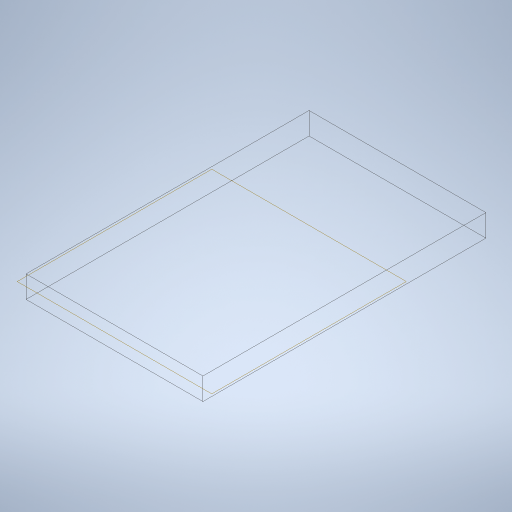
# Autodesk Inventor part: strain gauge v2
Saved by Autodesk Inventor 2024.2 (Build 282272000, 272)
## iProperties
Created: 2024-07-11
Part Number: strain gauge v2
Material: Generic
Document SubType Name: Modeling
Designer: Tom
Density: 1 g/cm^3
Appearance: Default
Author: Tom
Autodesk Inventor part; units mm, degrees
ref_plane "YZ Plane" through (0, 0, 0) normal (1, 0, 0) x (0, 1, 0)
ref_plane "XY Plane" through (0, 0, 0) normal (0, 0, 1) x (1, 0, 0)
sketch "Sketch1" plane through (0, 0, 0) normal (0, 1, 0) x (-1, 0, 0)
  line L0 (0, 0) -> (25.4, 0)
  line L1 (25.4, 0) -> (25.4, -38.1)
  line L2 (25.4, -38.1) -> (0, -38.1)
  line L3 (0, -38.1) -> (0, 0)
  dimension "d0" = 25.4
  dimension "d1" = 38.1
  constraints: 8 end point, 2 parallel, 1 horizontal, 1 perpendicular
  measures "d0" distance of L0.start L0.end
  measures "d1" distance of L0.end L1.end
extrude "Extrusion1" add sketch "Sketch1" along normal blind 3.175
ref_plane "Work Plane1" through (0, 1.5875, 0) normal (0, 1, 0) x (-1, 0, 0)
sketch "Sketch2" plane through (0, 1.5875, 0) normal (0, 1, 0) x (-1, 0, 0)
  line L0 (0, -2.1676) -> (22.225, -2.1676)
  line L1 (22.225, -2.1676) -> (22.225, -4.7076)
  line L2 (22.225, -4.7076) -> (2.852, -4.7076)
  line L3 (2.852, -4.7076) -> (2.852, -9.7876)
  line L4 (2.852, -9.7876) -> (22.225, -9.7876)
  line L5 (22.225, -9.7876) -> (22.225, -12.3276)
  line L6 (22.225, -12.3276) -> (2.852, -12.3276)
  line L7 (2.852, -12.3276) -> (2.852, -17.4076)
  line L8 (2.852, -17.4076) -> (22.225, -17.4076)
  line L9 (22.225, -17.4076) -> (22.225, -19.9476)
  line L10 (22.225, -19.9476) -> (2.852, -19.9476)
  line L11 (2.852, -19.9476) -> (2.852, -25.0276)
  line L12 (2.852, -25.0276) -> (22.225, -25.0276)
  line L13 (22.225, -25.0276) -> (22.225, -27.5676)
  line L14 (22.225, -27.5676) -> (2.3031, -27.5676)
  line L15 (2.3031, -27.5676) -> (2.3031, -32.6476)
  line L16 (2.3031, -32.6476) -> (22.225, -32.6476)
  line L17 (22.225, -32.6476) -> (22.225, -35.1876)
  line L18 (22.225, -35.1876) -> (0, -35.1876)
  line L19 (0, -2.1676) -> (0.606, -2.1676)
  point P0 (0, 0)
  point P1 (22.225, -3.4376)
  dimension "d5" = 2.54
  dimension "d6" = 2.54
  dimension "d7" = 2.54
  dimension "d8" = 2.54
  dimension "d9" = 5.08
  dimension "d10" = 5.08
  dimension "d11" = 5.08
  dimension "d12" = 22.225
  dimension "d13" = 19.373
  dimension "d15" = 5.08
  dimension "d16" = 2.54
  constraints: 40 end point, 12 perpendicular, 9 point on line, 3 horizontal, 1 midpoint, 1 vertical
  measures "d5" distance of L0.end L1.end
  measures "d6" distance of L4.end L5.end
  measures "d7" distance of L8.end L9.end
  measures "d8" distance of L12.end L13.end
  measures "d9" distance of L10.end L11.end
  measures "d10" distance of L6.end L7.end
  measures "d11" distance of L2.end L3.end
  measures "d12" distance of L0.start L0.end
  measures "d13" distance of L3.end L4.end
  measures "d15" distance of L14.end L15.end
  measures "d16" distance of L16.end L17.end
sketch "Sketch4" plane through (0, 0, 0) normal (1, 0, 0) x (0, 1, 0)
  circle A0 centre (1.5984, -1.4405) radius 0.889
  point P0 (0, 0)
  dimension "d17" = 1.778
  constraints: 1 centre point
  measures "d17" diameter of A0
sweep "Sweep1" [suppressed]
sketch "Sketch5" plane through (0, 0, -38.1) normal (0, 0, -1) x (-1, 0, 0)
  line L0 (0, 3.175) -> (25.4, 3.175) projected
  line L1 (0, 0) -> (25.4, 0) projected
  line L2 (0, 3.175) -> (25.4, 3.175)
  line L3 (25.4, 3.175) -> (25.4, 0)
  line L4 (25.4, 0) -> (0, 0)
  line L5 (0, 0) -> (0, 3.175)
  constraints: 8 end point, 2 parallel, 1 horizontal, 1 perpendicular
extrude "Extrusion2" add sketch "Sketch5" along normal blind 1.27
sketch "Sketch6" plane through (-25.4, 0, 0) normal (0, 0, 1) x (1, 0, 0)
  line L0 (0, 3.175) -> (25.4, 3.175) projected
  line L1 (0, 0) -> (25.4, 0) projected
  line L2 (0, 3.175) -> (25.4, 3.175)
  line L3 (25.4, 3.175) -> (25.4, 0)
  line L4 (25.4, 0) -> (0, 0)
  line L5 (0, 0) -> (0, 3.175)
  constraints: 8 end point, 2 parallel, 1 horizontal, 1 perpendicular
extrude "Extrusion3" add sketch "Sketch6" along normal blind 1.27
body "Solid1"
